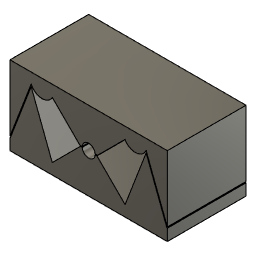
filaWelder v11 (Autodesk Fusion 360 design; units mm, degrees)
Autodesk Fusion 360 part; units mm, degrees
note: some values were not read from the file. Chosen so that the rebuilt part matches the saved one: which bodies a step acts on; which pieces of a blend or face edit are solid. Set by a fixed rule: which sketch regions a step uses.
sketch "Sketch1" plane through (0, 0, 0) normal (0, 0, 1) x (1, 0, 0)
  line L0 (10, 5) -> (-10, 5)
  line L1 (-10, 5) -> (-10, -5)
  line L2 (-10, -5) -> (10, -5)
  line L3 (10, -5) -> (10, 5)
  line L4 (10, 5) -> (-10, -5) construction
  line L5 (-10, 5) -> (10, -5) construction
  circle A0 centre (0, 0) radius 0.825
  circle A1 centre (0, 0) radius 1.075
  line L6 (-10, 0) -> (10, 0)
  line L7 (-1.075, 0) -> (-4.6105, 3.5355)
  line L8 (-4.6105, 3.5355) -> (-4.6105, 0)
  line L9 (-1.075, 0) -> (-4.6105, -3.5355)
  line L10 (-4.6105, -3.5355) -> (-4.6105, 0)
  line L11 (0, 5) -> (0, -5) construction
  line L12 (1.075, 0) -> (4.6105, 3.5355)
  line L13 (4.6105, 3.5355) -> (4.6105, 0)
  line L14 (4.6105, -3.5355) -> (4.6105, 0)
  line L15 (1.075, 0) -> (4.6105, -3.5355)
  dimension "d1" = 20
  dimension "d2" = 10
  dimension "d3" = 1.65
  dimension "d31" = 0.25
  dimension "d32" = 45
  dimension "d33" = 5
  constraint horizontal L0
  constraint perpendicular L0 L1
  constraint parallel L0 L2
  constraint parallel L1 L3
  constraint coincident L4 A0.centre
  constraint coincident L5 A0.centre
  constraint coincident A0.centre A1.centre
  constraint midpoint L1 L6.start
  constraint midpoint L3 L6.end
  constraint coincident A1 L7.start
  constraint coincident L6 L7.start
  constraint coincident L6 L8.end
  constraint perpendicular L6 L8
  constraint symmetric L6 L7.start L9.start
  constraint symmetric L6 L7.end L9.end
  constraint symmetric L6 L8.end L10.end
  constraint midpoint L0 L11.start
  constraint midpoint L2 L11.end
  constraint symmetric L7.start L11 L12.start
  constraint symmetric L7.end L11 L12.end
  constraint symmetric L8.end L11 L13.end
  constraint symmetric L9.end L11 L14.start
  measures "d1" distance of L1.end L2.end
  measures "d2" distance of L0.end L1.end
  measures "d3" diameter of A0
  measures "d32" angle of L6 L7
  measures "d33" distance of L7.start L7.end
extrude "Extrude1" add sketch "Sketch1" along normal mid plane 40 contours L0 L1 L3 A1 L6 L7 L8 L12 L13 | L1 L2 L3 A1 L6 L9 L10 L14 L15 | A0 A1 L6 | A0 A1 L6 makes body 1
sketch "Sketch2" plane through (0, 0, 20) normal (0, 0, 1) x (1, 0, 0)
  line L0 (4.6105, 3.5355) -> (10, 3.5355) construction
  line L1 (4.6105, -3.5355) -> (10, -3.5355) construction
  line L2 (4.6105, -3.5355) -> (1.075, 0) construction
  line L3 (1.075, 0) -> (0, 0) construction
  line L4 (4.6105, -3.5355) -> (7.3053, 3.5355) construction
  line L5 (7.3053, 3.5355) -> (10, -3.5355) construction
  line L6 (1.0543, -0.05) -> (0, -0.05)
  line L7 (4.6298, -3.6255) -> (1.0543, -0.05)
  line L8 (4.6298, -3.6255) -> (7.3053, 3.3951)
  line L9 (7.3053, 3.3951) -> (9.9533, -3.5533)
  line L10 (1.0957, 0.05) -> (0, 0.05)
  line L11 (4.5913, -3.4456) -> (1.0957, 0.05)
  line L12 (4.5913, -3.4456) -> (7.3053, 3.6759)
  line L13 (7.3053, 3.6759) -> (10.0467, -3.5177)
  line L14 (10.0467, -3.5177) -> (9.9533, -3.5533)
  line L15 (0, 0.8) -> (0, -0.7) construction
  line L16 (-4.6105, -3.5355) -> (-1.075, 0) construction
  line L17 (-1.0543, -0.05) -> (0, -0.05)
  line L18 (-4.5913, -3.4456) -> (-1.0957, 0.05)
  line L19 (-7.3053, 3.3951) -> (-9.9533, -3.5533)
  line L20 (-4.6298, -3.6255) -> (-7.3053, 3.3951)
  line L21 (-1.075, 0) -> (0, 0) construction
  line L22 (-7.3053, 3.6759) -> (-10.0467, -3.5177)
  line L23 (-10.0467, -3.5177) -> (-9.9533, -3.5533)
  line L24 (-7.3053, 3.5355) -> (-10, -3.5355) construction
  line L25 (-4.6105, -3.5355) -> (-10, -3.5355) construction
  line L26 (-4.6298, -3.6255) -> (-1.0543, -0.05)
  line L27 (-4.5913, -3.4456) -> (-7.3053, 3.6759)
  line L28 (-1.0957, 0.05) -> (0, 0.05)
  line L29 (-4.6105, -3.5355) -> (-7.3053, 3.5355) construction
  line L30 (-4.6105, 3.5355) -> (-10, 3.5355) construction
  point P0 (4.6105, 3.5355)
  point P1 (4.6105, -3.5355)
  point P2 (1.075, 0)
  point P3 (-4.6105, -3.5355)
  point P4 (-1.075, 0)
  point P5 (-4.6105, 3.5355)
  point P6 (0, -0.7)
  point P7 (0, 0.8)
  dimension "d34" = 0.05
  dimension "d35" = 0.05
  constraint coincident P0 L0.start
  constraint horizontal L0
  constraint coincident P1 L1.start
  constraint parallel L0 L1
  constraint coincident P2 L2.end
  constraint coincident L3.end L21.end
  constraint midpoint L0 L4.end
  constraint perpendicular L9 L14
  constraint perpendicular L10 L15
  constraint symmetric L3.end L15 L21.end
  constraint symmetric P0 L15 P5
  constraint symmetric L0.end L15 L30.end
  constraint symmetric P1 L15 L16.start
  constraint symmetric L1.end L15 L24.end
  constraint symmetric P1 L15 P3
  constraint symmetric P2 L15 P4
  constraint symmetric L4.end L15 L24.start
  constraint symmetric L6.start L15 L17.start
  constraint symmetric L6.end L15 L17.end
  constraint symmetric L7.start L15 L20.start
  constraint symmetric L8.end L15 L19.start
  constraint symmetric L9.end L15 L19.end
  constraint symmetric L10.start L15 L18.end
  constraint symmetric L10.end L15 L28.end
  constraint symmetric L11.start L15 L18.start
  constraint symmetric L12.end L15 L22.start
  constraint symmetric L13.end L15 L22.end
  constraint symmetric P7 L15 L15.start
  constraint symmetric P6 L15 L15.end
split "Split1" by curves path "Sketch2" along L6 L7 L8 L9 L14 L13 L12 L11 L10 L28 L18 L27 L22 L23 L19 L20 L26 L17 bodies 1 makes body 2 at (3.3333, -5, 6.6667) makes body 3 at (-3.3333, 5, 6.6667) makes body 4 at (2.2535, -1.1785, 6.6667)
ref_plane "WorkPlane2" through (0, 5, 0) normal (0, 1, 0) x (-1, 0, 0)
sketch "Sketch3" plane through (0, 5, 0) normal (0, 1, 0) x (1, 0, 0)
  line L0 (-20, 20) -> (20, 20)
  line L1 (20, 20) -> (20, 5)
  line L2 (20, 5) -> (-20, 5)
  line L3 (-20, 5) -> (-20, 20)
  line L4 (-20, -5) -> (20, -5)
  line L5 (20, -5) -> (20, -20)
  line L6 (20, -20) -> (-20, -20)
  line L7 (-20, -20) -> (-20, -5)
  dimension "d19" = 10
  dimension "d20" = 40
  constraint horizontal L0
  constraint vertical L1
  constraint horizontal L2
  constraint vertical L3
  constraint horizontal L4
  constraint vertical L5
  constraint horizontal L6
  constraint vertical L7
  measures "d19" distance of L2 L4
  measures "d20" distance of L0 L6
extrude "Extrude4" cut sketch "Sketch3" against normal blind 11 bodies 3 2
fillet "Fillet1" radius 1.5 2 edges at (-4.6105, -3.3951, 0) (4.6105, -3.3951, 0) on bodies 3
hidden bodies 1 4
